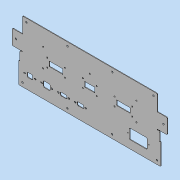
# Autodesk Inventor part: Back_Mount_Flat
Saved by Autodesk Inventor 2020 (Build 240168000, 168)
## iProperties
Created: 2021-06-14
Part Number: Back_Mount_Flat
Material: Generic
Document SubType Name: Modeling
Designer: magnarecta
Density: 1 g/cm^3
Appearance: Default
Author: magnarecta
Autodesk Inventor part; units mm, degrees
ref_plane "YZ Plane" through (0, 0, 0) normal (1, 0, 0) x (0, 1, 0)
ref_plane "XZ Plane" through (0, 0, 0) normal (0, 1, 0) x (-1, 0, 0)
ref_plane "XY Plane" through (0, 0, 0) normal (0, 0, 1) x (1, 0, 0)
sketch "スケッチ1" plane through (0, 0, 0) normal (0, 0, 1) x (1, 0, 0)
  circle A0 centre (385.2191, 102.2191) radius 2.25
  circle A1 centre (18.4, 154.4382) radius 2.25
  circle A2 centre (248.4, 154.4382) radius 2.25
  circle A3 centre (358.4, 154.4382) radius 2.25
  circle A4 centre (128.4, 154.4382) radius 2.25
  circle A5 centre (301.5, 77.7191) radius 1.75
  circle A6 centre (254.5, 100.7191) radius 1.75
  circle A7 centre (254.5, 77.7191) radius 1.75
  circle A8 centre (301.5, 100.7191) radius 1.75
  circle A9 centre (313, 120.2191) radius 1.75
  circle A10 centre (63, 70.2191) radius 1.75
  circle A11 centre (63, 120.2191) radius 1.75
  circle A12 centre (313, 70.2191) radius 1.75
  circle A13 centre (188, 120.2191) radius 1.75
  circle A14 centre (74.5, 77.7191) radius 1.75
  circle A15 centre (121.5, 100.7191) radius 1.75
  circle A16 centre (121.5, 77.7191) radius 1.75
  circle A17 centre (74.5, 100.7191) radius 1.75
  line L0 (116.5, 94.7191) -> (116.5, 83.7191)
  arc A18 (115.5, 82.7191) -> (116.5, 83.7191) centre (115.5, 83.7191) ccw
  line L1 (115.5, 82.7191) -> (80.5, 82.7191)
  arc A19 (79.5, 83.7191) -> (80.5, 82.7191) centre (80.5, 83.7191) ccw
  line L2 (79.5, 83.7191) -> (79.5, 94.7191)
  arc A20 (80.5, 95.7191) -> (79.5, 94.7191) centre (80.5, 94.7191) ccw
  line L3 (80.5, 95.7191) -> (115.5, 95.7191)
  arc A21 (116.5, 94.7191) -> (115.5, 95.7191) centre (115.5, 94.7191) ccw
  line L4 (260.5, 95.7191) -> (295.5, 95.7191)
  arc A22 (296.5, 94.7191) -> (295.5, 95.7191) centre (295.5, 94.7191) ccw
  line L5 (296.5, 94.7191) -> (296.5, 83.7191)
  arc A23 (295.5, 82.7191) -> (296.5, 83.7191) centre (295.5, 83.7191) ccw
  line L6 (295.5, 82.7191) -> (260.5, 82.7191)
  arc A24 (259.5, 83.7191) -> (260.5, 82.7191) centre (260.5, 83.7191) ccw
  line L7 (259.5, 83.7191) -> (259.5, 94.7191)
  arc A25 (260.5, 95.7191) -> (259.5, 94.7191) centre (260.5, 94.7191) ccw
  circle A26 centre (206.5, 77.7191) radius 1.75
  circle A27 centre (169.5, 100.7191) radius 1.75
  circle A28 centre (169.5, 77.7191) radius 1.75
  circle A29 centre (206.5, 100.7191) radius 1.75
  line L8 (175.5, 95.7191) -> (200.5, 95.7191)
  arc A30 (201.5, 94.7191) -> (200.5, 95.7191) centre (200.5, 94.7191) ccw
  line L9 (201.5, 94.7191) -> (201.5, 83.7191)
  arc A31 (200.5, 82.7191) -> (201.5, 83.7191) centre (200.5, 83.7191) ccw
  line L10 (200.5, 82.7191) -> (175.5, 82.7191)
  arc A32 (174.5, 83.7191) -> (175.5, 82.7191) centre (175.5, 83.7191) ccw
  line L11 (174.5, 83.7191) -> (174.5, 94.7191)
  arc A33 (175.5, 95.7191) -> (174.5, 94.7191) centre (175.5, 94.7191) ccw
  circle A34 centre (128, 10) radius 2.25
  circle A35 centre (8, 10) radius 2.25
  circle A36 centre (368, 10) radius 2.25
  circle A37 centre (248, 10) radius 2.25
  arc A38 (58, 36.6) -> (58, 33.4) centre (58, 35) ccw
  line L12 (58, 36.6) -> (60, 36.6)
  arc A39 (60, 33.4) -> (60, 36.6) centre (60, 35) ccw
  line L13 (60, 33.4) -> (58, 33.4)
  arc A40 (150, 33.4) -> (150, 36.6) centre (150, 35) ccw
  line L14 (150, 33.4) -> (148, 33.4)
  arc A41 (148, 36.6) -> (148, 33.4) centre (148, 35) ccw
  line L15 (148, 36.6) -> (150, 36.6)
  line L16 (131, 36.6) -> (133, 36.6)
  arc A42 (133, 33.4) -> (133, 36.6) centre (133, 35) ccw
  line L17 (133, 33.4) -> (131, 33.4)
  arc A43 (131, 36.6) -> (131, 33.4) centre (131, 35) ccw
  arc A44 (41, 36.6) -> (41, 33.4) centre (41, 35) ccw
  line L18 (41, 36.6) -> (43, 36.6)
  arc A45 (43, 33.4) -> (43, 36.6) centre (43, 35) ccw
  line L19 (43, 33.4) -> (41, 33.4)
  arc A46 (86, 36.6) -> (86, 33.4) centre (86, 35) ccw
  line L20 (86, 36.6) -> (88, 36.6)
  arc A47 (88, 33.4) -> (88, 36.6) centre (88, 35) ccw
  line L21 (88, 33.4) -> (86, 33.4)
  line L22 (176, 36.6) -> (178, 36.6)
  arc A48 (178, 33.4) -> (178, 36.6) centre (178, 35) ccw
  line L23 (178, 33.4) -> (176, 33.4)
  arc A49 (176, 36.6) -> (176, 33.4) centre (176, 35) ccw
  arc A50 (103, 36.6) -> (103, 33.4) centre (103, 35) ccw
  line L24 (103, 36.6) -> (105, 36.6)
  arc A51 (105, 33.4) -> (105, 36.6) centre (105, 35) ccw
  line L25 (105, 33.4) -> (103, 33.4)
  arc A52 (15, 33.4) -> (15, 36.6) centre (15, 35) ccw
  line L26 (15, 33.4) -> (13, 33.4)
  arc A53 (13, 36.6) -> (13, 33.4) centre (13, 35) ccw
  line L27 (13, 36.6) -> (15, 36.6)
  line L28 (171.5, 37.5) -> (171.5, 32.5)
  arc A54 (169.5, 30.5) -> (171.5, 32.5) centre (169.5, 32.5) ccw
  line L29 (169.5, 30.5) -> (156.5, 30.5)
  arc A55 (154.5, 32.5) -> (156.5, 30.5) centre (156.5, 32.5) ccw
  line L30 (154.5, 32.5) -> (154.5, 37.5)
  arc A56 (156.5, 39.5) -> (154.5, 37.5) centre (156.5, 37.5) ccw
  line L31 (156.5, 39.5) -> (169.5, 39.5)
  arc A57 (171.5, 37.5) -> (169.5, 39.5) centre (169.5, 37.5) ccw
  line L32 (109.5, 32.5) -> (109.5, 37.5)
  arc A58 (111.5, 39.5) -> (109.5, 37.5) centre (111.5, 37.5) ccw
  line L33 (111.5, 39.5) -> (124.5, 39.5)
  arc A59 (126.5, 37.5) -> (124.5, 39.5) centre (124.5, 37.5) ccw
  line L34 (126.5, 37.5) -> (126.5, 32.5)
  arc A60 (124.5, 30.5) -> (126.5, 32.5) centre (124.5, 32.5) ccw
  line L35 (124.5, 30.5) -> (111.5, 30.5)
  arc A61 (109.5, 32.5) -> (111.5, 30.5) centre (111.5, 32.5) ccw
  line L36 (82, 40.5) -> (82, 29.5)
  arc A62 (80, 27.5) -> (82, 29.5) centre (80, 29.5) ccw
  line L37 (80, 27.5) -> (66, 27.5)
  arc A63 (64, 29.5) -> (66, 27.5) centre (66, 29.5) ccw
  line L38 (64, 29.5) -> (64, 40.5)
  arc A64 (66, 42.5) -> (64, 40.5) centre (66, 40.5) ccw
  line L39 (66, 42.5) -> (80, 42.5)
  arc A65 (82, 40.5) -> (80, 42.5) centre (80, 40.5) ccw
  line L40 (33, 29) -> (23, 29)
  arc A66 (21, 31) -> (23, 29) centre (23, 31) ccw
  line L41 (21, 31) -> (21, 39)
  arc A67 (23, 41) -> (21, 39) centre (23, 39) ccw
  line L42 (23, 41) -> (33, 41)
  arc A68 (35, 39) -> (33, 41) centre (33, 39) ccw
  line L43 (35, 39) -> (35, 31)
  arc A69 (33, 29) -> (35, 31) centre (33, 31) ccw
  circle A70 centre (290, 35) radius 1.2295
  circle A71 centre (346, 35) radius 1.2295
  line L44 (341.5, 46.5) -> (341.5, 23.5)
  arc A72 (339.5, 21.5) -> (341.5, 23.5) centre (339.5, 23.5) ccw
  line L45 (339.5, 21.5) -> (296.5, 21.5)
  arc A73 (294.5, 23.5) -> (296.5, 21.5) centre (296.5, 23.5) ccw
  line L46 (294.5, 23.5) -> (294.5, 46.5)
  arc A74 (296.5, 48.5) -> (294.5, 46.5) centre (296.5, 46.5) ccw
  line L47 (296.5, 48.5) -> (339.5, 48.5)
  arc A75 (341.5, 46.5) -> (339.5, 48.5) centre (339.5, 46.5) ccw
  circle A76 centre (-9.2191, 102.2191) radius 2.25
  arc A77 (-17.2191, 122.2191) -> (-19.2191, 120.2191) centre (-17.2191, 120.2191) ccw
  line L48 (-19.2191, 84.2191) -> (-19.2191, 120.2191)
  arc A78 (-19.2191, 84.2191) -> (-17.2191, 82.2191) centre (-17.2191, 84.2191) ccw
  line L49 (-17.2191, 82.2191) -> (7.2, 82.2191)
  line L50 (7.2, 82.2191) -> (7.2, 80.2191)
  line L51 (7.2, 80.2191) -> (3.2, 80.2191)
  arc A79 (3.2, 80.2191) -> (1.2, 78.2191) centre (3.2, 78.2191) ccw
  line L52 (1.2, 78.2191) -> (1.2, 56.8)
  line L53 (1.2, 56.8) -> (0, 56.8)
  arc A80 (0, 56.8) -> (-2, 54.8) centre (0, 54.8) ccw
  line L54 (-2, 2) -> (-2, 54.8)
  arc A81 (-2, 2) -> (0, 0) centre (0, 2) ccw
  line L55 (376, 0) -> (0, 0)
  arc A82 (376, 0) -> (378, 2) centre (376, 2) ccw
  line L56 (378, 54.8) -> (378, 2)
  arc A83 (378, 54.8) -> (376, 56.8) centre (376, 54.8) ccw
  line L57 (376, 56.8) -> (374.8, 56.8)
  line L58 (374.8, 56.8) -> (374.8, 78.2191)
  arc A84 (374.8, 78.2191) -> (372.8, 80.2191) centre (372.8, 78.2191) ccw
  line L59 (372.8, 80.2191) -> (368.8, 80.2191)
  line L60 (368.8, 80.2191) -> (368.8, 82.2191)
  line L61 (368.8, 82.2191) -> (393.2191, 82.2191)
  arc A85 (393.2191, 82.2191) -> (395.2191, 84.2191) centre (393.2191, 84.2191) ccw
  line L62 (395.2191, 120.2191) -> (395.2191, 84.2191)
  arc A86 (395.2191, 120.2191) -> (393.2191, 122.2191) centre (393.2191, 120.2191) ccw
  line L63 (393.2191, 122.2191) -> (368.4, 122.2191)
  line L64 (368.4, 122.2191) -> (368.4, 162.4382)
  arc A87 (368.4, 162.4382) -> (366.4, 164.4382) centre (366.4, 162.4382) ccw
  line L65 (366.4, 164.4382) -> (10.4, 164.4382)
  arc A88 (10.4, 164.4382) -> (8.4, 162.4382) centre (10.4, 162.4382) ccw
  line L66 (8.4, 162.4382) -> (8.4, 122.2191)
  line L67 (8.4, 122.2191) -> (-17.2191, 122.2191)
  constraints: 136 end point, 120 point on circle, 89 centre point
extrude "押し出し1" add sketch "スケッチ1" along normal blind 1.6
